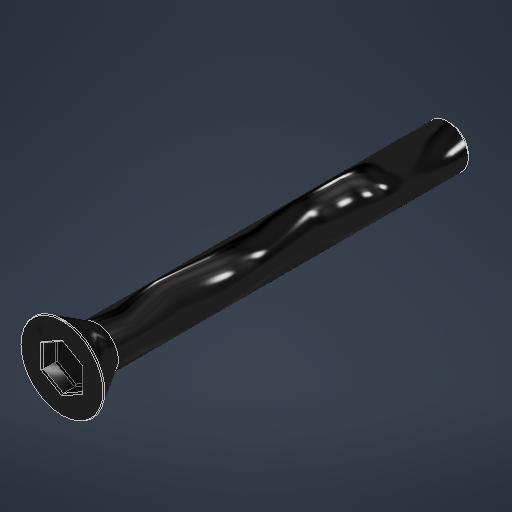
# Autodesk Inventor part: M3_Screw
Saved by Autodesk Inventor 2026 (Build 300175000, 175)
## iProperties
Created: 2025-11-29
Part Number: M3_Screw
Material: Steel
Document SubType Name: Modeling
Designer: pochi
Density: 7.85 g/cm^3
Appearance: Black
Mass: 1.65636 g
Surface Area: 3.17576 cm^2
Volume: 0.211001 cm^3
Author: pochi
Autodesk Inventor part; units mm, degrees
ref_plane "YZ Plane" through (0, 0, 0) normal (1, 0, 0) x (0, 1, 0)
ref_plane "XZ Plane" through (0, 0, 0) normal (0, 1, 0) x (-1, 0, 0)
ref_plane "XY Plane" through (0, 0, 0) normal (0, 0, 1) x (1, 0, 0)
sketch "Sketch1" plane through (0, 0, 0) normal (0, 0, 1) x (1, 0, 0)
  circle A0 centre (0, 0) radius 1.5
  dimension "d0" = 3
  constraints: 1 centre point, 1 coincident
  measures "d0" diameter of A0
extrude "Extrusion1" add sketch "Sketch1" against normal blind 25
sketch "Sketch2" plane through (0, 0, 0) normal (0, 0, 1) x (1, 0, 0)
  circle A0 centre (0, 0) radius 1.5 projected
  circle A1 centre (0, 0) radius 3
  dimension "d3" = 6
  constraints: 1 centre point, 1 coincident
  measures "d3" diameter of A1
extrude "Extrusion2" add sketch "Sketch2" along normal blind 2.5 contours A0 | A1
draft "FaceDraft1" angle 31 pull direction (0, 0, -1) faces at (2.9612, -0.4812, 1.6667) fixed edges at (-3, 0, 2.5)
chamfer "Chamfer1" distance 0.2 angle 45 1 edges at (-1.5, 0, -25)
sketch "Sketch3" plane through (0, 0, 2.5) normal (0, 0, 1) x (1, 0, 0)
  circle A0 centre (0, 0) radius 3 construction
  circle A1 centre (0, 0) radius 1.6 construction
  line L0 (0, -1.6) -> (-1.3856, -0.8)
  line L1 (-1.3856, -0.8) -> (-1.3856, 0.8)
  line L2 (-1.3856, 0.8) -> (0, 1.6)
  line L3 (0, 1.6) -> (1.3856, 0.8)
  line L4 (1.3856, 0.8) -> (1.3856, -0.8)
  line L5 (1.3856, -0.8) -> (0, -1.6)
  dimension "d10" = 1.4
  constraints: 12 end point, 1 coincident, 1 vertical alignment, 15 other
extrude "Extrusion3" cut sketch "Sketch3" against normal blind 1
chamfer "Chamfer2" distance 0.1 angle 45 13 edges at (0.6928, -1.2, 2.5) (-0.6928, -1.2, 2.5) (-1.3856, 0, 2.5) (-0.6928, 1.2, 2.5) (0.6928, 1.2, 2.5) (1.3856, 0, 2.5) (-3, 0, 2.5) (0.6928, 1.2, 1.5) (1.3856, 0, 1.5) (-0.6928, 1.2, 1.5) (0.6928, -1.2, 1.5) (-0.6928, -1.2, 1.5) (-1.3856, 0, 1.5)
body "Solid1"
